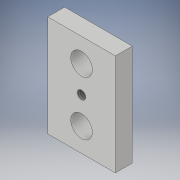
# Autodesk Inventor part: ShoulderScrewHolderSlide
Saved by Autodesk Inventor 2017 (Build 210142000, 142)
## iProperties
Created: 2017-12-26
Part Number: ShoulderScrewHolderSlide
Material: Generic
Document SubType Name: Modeling
Designer: User
Density: 1 g/cm^3
Appearance: Default
Author: User
Autodesk Inventor part; units mm, degrees
ref_plane "YZ Plane" through (0, 0, 0) normal (1, 0, 0) x (0, 1, 0)
ref_plane "XZ Plane" through (0, 0, 0) normal (0, 1, 0) x (-1, 0, 0)
ref_plane "XY Plane" through (0, 0, 0) normal (0, 0, 1) x (1, 0, 0)
sketch "Sketch1" plane through (0, 0, 0) normal (0, 0, 1) x (1, 0, 0)
  line L0 (0, 0) -> (12.7, 0)
  line L1 (12.7, 0) -> (12.7, 19.05)
  line L2 (12.7, 19.05) -> (0, 19.05)
  line L3 (0, 19.05) -> (0, 0)
  dimension "d0" = 12.7
  dimension "d1" = 19.05
  constraints: 8 end point, 2 parallel, 1 horizontal, 1 perpendicular
  measures "d0" distance of L2.end L1.end
  measures "d1" distance of L1.end L0.end
extrude "Extrusion1" add sketch "Sketch1" along normal blind 3.175
sketch "Sketch2" plane through (0, 0, 3.175) normal (0, 0, 1) x (1, 0, 0)
  line L0 (12.7, 19.05) -> (0, 19.05) projected
  line L1 (6.35, 19.05) -> (6.35, 14.605)
  circle A0 centre (6.35, 14.605) radius 2.032
  line L2 (0, 19.05) -> (0, 0) projected
  line L3 (0, 9.525) -> (6.35, 9.525)
  line L4 (0, 0) -> (12.7, 0) projected
  line L5 (6.35, 0) -> (6.35, 4.445)
  dimension "d4" = 4.445
  dimension "d5" = 4.064
  dimension "d15" = 4.445
  constraints: 6 end point, 3 coincident, 3 midpoint, 2 vertical, 1 centre point, 1 horizontal
  measures "d4" distance of L1.start L1.end
  measures "d5" diameter of A0
  measures "d15" distance of L5.start L5.end
hole "Hole1" at (6.35, 9.525, 3.175) direction (0, 0, -1) diameter 1.5748 end through all
extrude "Extrusion2" cut sketch "Sketch2" against normal blind 25.4
hole "Hole2" at (6.35, 4.445, 3.175) direction (0, 0, -1) diameter 4.064 end through all
body "Solid1"
